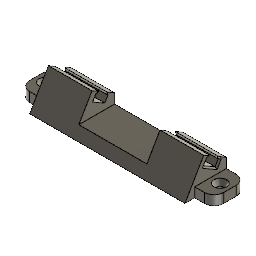
dsi-base-angled (Autodesk Fusion 360 design; units mm, degrees)
Autodesk Fusion 360 part; units mm, degrees
sketch "Sketch1" plane through (0, 0, 0) normal (1, 0, 0) x (0, 1, 0)
  line L0 (-1.0104, 16.75) -> (-10.681, 0)
  line L1 (-10.681, 0) -> (10.681, 0)
  line L2 (10.681, 0) -> (10.681, 10)
  line L3 (10.681, 10) -> (-1.0104, 16.75)
  line L4 (1.5877, 15.25) -> (-0.5373, 11.5694)
  line L5 (-0.5373, 11.5694) -> (5.5249, 8.0694)
  line L6 (5.5249, 8.0694) -> (7.6499, 11.75)
  line L7 (7.6499, 11.75) -> (1.5877, 15.25) construction
  line L8 (5.5249, 8.0694) -> (-0.5373, 8.0694) construction
  line L9 (-0.5373, 8.0694) -> (-0.5373, 11.5694) construction
  line L10 (10.681, 7.5463) -> (6.5874, 9.9097) construction
  line L11 (0.5252, 13.4097) -> (-2.0729, 14.9097) construction
  line L12 (7.0249, 10.6675) -> (6.5674, 12.375) construction
  line L13 (0.9627, 14.1675) -> (2.6702, 14.625) construction
  dimension "d1" = 30
  dimension "d2" = 7
  dimension "d5" = 10
  dimension "d6" = 3.5
  dimension "d7" = 60
  dimension "d24" = 3
  dimension "d34" = 3
  dimension "d35" = 1.25
  dimension "d36" = 1.25
  dimension "d38" = 45
  constraint horizontal L1
  constraint midpoint origin L1
  constraint perpendicular L4 L5
  constraint perpendicular L5 L6
  constraint perpendicular L6 L7
  constraint horizontal L8
  constraint vertical L9
  constraint parallel L3 L7
  constraint coincident L3 L4.start
  constraint vertical L2
  constraint coincident L2 L10.start
  constraint midpoint L6 L10.end
  constraint midpoint L4 L11.start
  constraint coincident L0 L11.end
  constraint perpendicular L4 L11
  constraint parallel L10 L11
  constraint coincident L6 L12.start
  constraint coincident L7 L12.end
  constraint coincident L4 L13.start
  constraint coincident L7 L13.end
  constraint equal L12 L13
  measures "d1" angle of L5 L8
  measures "d2" distance of L4.start L6.end
  measures "d5" vertical distance of L1.end L2.end
  measures "d6" distance of L2.end L6.end
  measures "d7" angle of L0 L1
  measures "d24" distance of L11.start L11.end
  measures "d34" distance of L5.end L12.start
  measures "d35" distance of L6.end L12.end
  measures "d36" distance of L4.start L13.end
  measures "d38" angle of L6 L12
extrude "Extrude1" add sketch "Sketch1" along normal mid plane 80
sketch "Sketch3" plane through (0, 0, 0) normal (0, 0, 1) x (1, 0, 0)
  line L0 (40, -10.681) -> (40, 10.681)
  line L1 (40, 10.681) -> (45, 10.681)
  line L2 (50, 5.681) -> (50, -0.681)
  line L3 (45, -5.681) -> (40, -5.681)
  line L4 (40, -5.681) -> (40, 10.681)
  arc A0 (50, 5.681) -> (45, 10.681) centre (45, 5.681) ccw
  arc A1 (45, -5.681) -> (50, -0.681) centre (45, -0.681) ccw
  dimension "d11" = 5
  dimension "d12" = 10
  dimension "d15" = 5
  constraint horizontal L1
  constraint vertical L2
  constraint horizontal L3
  constraint vertical L4
  constraint coincident L0.end L1.start
  constraint tangent L1 A0
  constraint tangent L2 A0
  constraint tangent L2 A1
  constraint tangent L3 A1
  constraint equal A0 A1
  measures "d11" radius of A0
  measures "d12" horizontal distance of L0.end L2.start
  measures "d15" distance of L0.start L3.end
extrude "Extrude2" add sketch "Sketch3" along normal blind 5
sketch "Sketch4" plane through (0, 0, 5) normal (0, 0, 1) x (-1, 0, 0)
  line L0 (-40, 5.681) -> (-45, 5.681)
  arc A0 (-45, 5.681) -> (-50, 0.681) centre (-45, 0.681) ccw
  line L1 (-50, 0.681) -> (-50, -5.681)
  arc A1 (-50, -5.681) -> (-45, -10.681) centre (-45, -5.681) ccw
  line L2 (-45, -10.681) -> (-40, -10.681)
  line L3 (-40, -10.681) -> (-40, 5.681)
  circle A2 centre (-45, -2.5) radius 1.75
  line L4 (-45, -10.681) -> (-45, 5.681) construction
  line L5 (-40, -10.681) -> (-50, -10.681) construction
  line L6 (-50, -5.681) -> (-50, -10.681) construction
  dimension "d16" = 3.5
  constraint midpoint A2.centre L4
  constraint coincident L0 A0.start
  constraint coincident L2 A1.end
  constraint vertical L4
  constraint coincident L2.end L3.start
  constraint perpendicular L3 L5
  constraint coincident L1.end A1.start
  constraint vertical L6
  constraint midpoint A1.end L5
  measures "d16" diameter of A2
extrude "Extrude3" cut sketch "Sketch4" against normal up to surface (5 mm away) contours A2
chamfer "Chamfer1" distance 1.5 angle 60 1 edges at (46.6316, 1.8672, 5) measured on face at (43.0417, -3.4592, 5)
mirror "Mirror1" about plane through (0, 0, 0) normal (1, 0, 0) of "Extrude2", "Extrude3", "Chamfer1"
sketch "Sketch5" plane through (40, 0, 0) normal (1, 0, 0) x (0, 1, 0)
  line L0 (-5.681, 0) -> (-5.681, 5)
  line L1 (-5.681, 5) -> (10.681, 5)
  line L2 (10.681, 5) -> (10.681, 10)
  line L3 (10.681, 10) -> (-1.0104, 16.75)
  line L4 (-1.0104, 16.75) -> (-10.681, 0)
  line L5 (-10.681, 0) -> (-5.681, 0)
  line L6 (1.5877, 15.25) -> (-0.5373, 11.5694) construction
  line L7 (-0.5373, 11.5694) -> (5.5249, 8.0694) construction
  line L8 (5.5249, 8.0694) -> (7.6499, 11.75) construction
  line L9 (1.5011, 15.3) -> (-0.6739, 11.5328)
  line L10 (-0.6739, 11.5328) -> (5.5615, 7.9328)
  line L11 (5.5615, 7.9328) -> (7.7365, 11.7)
  line L12 (0.9261, 14.3041) -> (2.497, 14.725)
  line L13 (7.1615, 10.7041) -> (6.7406, 12.275)
  dimension "d25" = 0.1
  dimension "d26" = 45
  dimension "d27" = 1.15
  dimension "d28" = 1.15
  constraint coincident L9 L12.start
  constraint coincident L3 L12.end
  constraint coincident L11 L13.start
  constraint coincident L3 L13.end
  constraint coincident L3 L9.start
  constraint equal L12 L13
  constraint coincident L3 L11.end
  measures "d26" angle of L9 L12
  measures "d27" distance of L9.start L12.end
  measures "d28" distance of L11.end L13.end
extrude "Extrude4" cut sketch "Sketch5" against normal up to surface (80 mm away) contours L3 L9 L10 L11 L12 L13
sketch "Sketch6" plane through (0, 0, 0) normal (0, 1, 0) x (1, 0, 0)
  line L0 (-40, -16.75) -> (40, -16.75)
  line L1 (-17.5, -16.75) -> (17.5, -16.75)
  line L2 (17.5, -16.75) -> (17.5, -5)
  line L3 (17.5, -5) -> (-17.5, -5)
  line L4 (-17.5, -5) -> (-17.5, -16.75)
  line L5 (40, -5) -> (45, -5)
  dimension "d32" = 35
  constraint horizontal L1
  constraint vertical L2
  constraint horizontal L3
  constraint vertical L4
  constraint coincident L0 L1.start
  constraint midpoint L0 L1
  constraint coincident L3 L5.start
  measures "d32" distance of L2.end L3.end
extrude "Extrude5" cut sketch "Sketch6" along normal through all and the other way through all
chamfer "Chamfer2" distance 0.75 angle 45 6 edges at (40, 0.1261, 12.9184) (40, 2.4438, 9.7328) (40, 6.3615, 9.3184) (-40, 2.4438, 9.7328) (-40, 0.1261, 12.9184) (-40, 6.3615, 9.3184)
chamfer "Chamfer3" distance 0.75 angle 45 4 edges at (40, 1.1993, 14.3773) (40, 7.0883, 10.9773) (-40, 7.0883, 10.9773) (-40, 1.1993, 14.3773)
